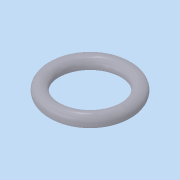
# Autodesk Inventor part: CoilSpring
Saved by Autodesk Inventor 2017 (Build 210142000, 142)
## iProperties
Created: 2016-10-13
Part Number: CoilSpring
Material: Generic
Document SubType Name: Modeling
Designer: techn
Density: 1 g/cm^3
Appearance: Weld - Stainless Steel
Author: techn
Autodesk Inventor part; units mm, degrees
ref_plane "YZ Plane" through (0, 0, 0) normal (1, 0, 0) x (0, 1, 0)
ref_plane "XZ Plane" through (0, 0, 0) normal (0, 1, 0) x (-1, 0, 0)
ref_plane "XY Plane" through (0, 0, 0) normal (0, 0, 1) x (1, 0, 0)
sketch "Sketch3" plane through (0, 0, 0) normal (1, 0, 0) x (0, 1, 0)
  circle A0 centre (0, 0) radius 0.635
  line L0 (0, -3.524) -> (5.0277, -3.524)
  dimension "d2" = 1.27
  dimension "d3" = 3.524
  constraints: 2 end point, 1 centre point, 1 coincident, 1 horizontal
  measures "d2" diameter of A0
  measures "d3" distance from line of L0 point (0, 0)
revolve "Revolution1" add sketch "Sketch3" angle 360 about axis through (0, 0, -3.524) along (0, 1, 0)
body "Solid1"
